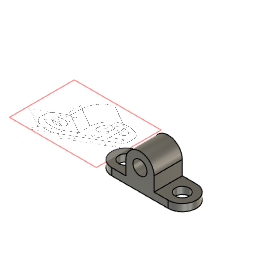
A4 v1 (Autodesk Fusion 360 design; units mm, degrees)
Autodesk Fusion 360 part; units mm, degrees
sketch "base" plane through (0, 0, 0) normal (0, 0, 1) x (1, 0, 0)
  line L0 (82.8311, -45.2427) -> (162.8311, -45.2427)
  line L1 (162.8311, -5.2427) -> (82.8311, -5.2427)
  line L2 (82.8311, -45.2427) -> (102.8311, -45.2427)
  line L3 (162.8311, -45.2427) -> (142.8311, -45.2427)
  circle A0 centre (82.8311, -25.2427) radius 10
  circle A1 centre (82.8311, -25.2427) radius 20
  line L4 (122.8311, -5.2427) -> (122.8311, -45.2427) construction
  circle A2 centre (162.8311, -25.2427) radius 20
  circle A3 centre (162.8311, -25.2427) radius 10
  line L5 (102.8311, -45.2427) -> (102.8311, -5.2427)
  line L6 (142.8311, -45.2427) -> (142.8311, -5.2427)
  dimension "d1" = 80
  dimension "d2" = 20
  dimension "d3" = 20
  dimension "d4" = 20
  dimension "d5" = 40
  constraint horizontal L0
  constraint horizontal L1
  constraint concentric A0 A1
  constraint tangent L1 A1
  constraint midpoint L1 L4.start
  constraint midpoint L0 L4.end
  constraint symmetric A0 L4 A3
  constraint symmetric A1 L4 A2
  constraint coincident L1 L5.end
  constraint perpendicular L1 L5
  constraint coincident L1 L6.end
  constraint perpendicular L1 L6
  measures "d1" distance of L0.start L0.end
  measures "d2" distance of L0.start L2.end
  measures "d3" distance of L0.end L3.end
  measures "d4" diameter of A0
  measures "d5" diameter of A1
extrude "Extrude1" add sketch "base" along normal blind 30 contours L0 L1 L5 L6
extrude "Extrude2" add sketch "base" along normal blind 10 contours L0 L2 A1 L5 | A1 | L1 A1 L5 | L0 L3 A2 L6 | A2 | L1 A2 L6
sketch "hole" plane through (0, -45.2427, 0) normal (0, -1, 0) x (1, 0, 0)
  line L0 (82.8311, 0) -> (162.8311, 0)
  line L1 (162.8311, 0) -> (162.8311, 10)
  line L2 (162.8311, 10) -> (142.8311, 10)
  line L3 (142.8311, 10) -> (142.8311, 30)
  line L4 (142.8311, 30) -> (102.8311, 30)
  line L5 (102.8311, 30) -> (102.8311, 10)
  line L6 (102.8311, 10) -> (82.8311, 10)
  line L7 (82.8311, 10) -> (82.8311, 0)
  circle A0 centre (122.8311, 30) radius 10
  circle A1 centre (122.8311, 30) radius 20
  dimension "d10" = 20
  dimension "d11" = 40
  constraint midpoint L4 A0.centre
  constraint concentric A0 A1
  measures "d10" diameter of A0
  measures "d11" diameter of A1
extrude "Extrude3" add sketch "hole" against normal blind 40 contours L4 A0 A1 picked at (111.3439, 42.0139)
extrude "Extrude4" cut sketch "hole" against normal blind 40 contours L4 A0 picked at (121.8402, 23.4262)
